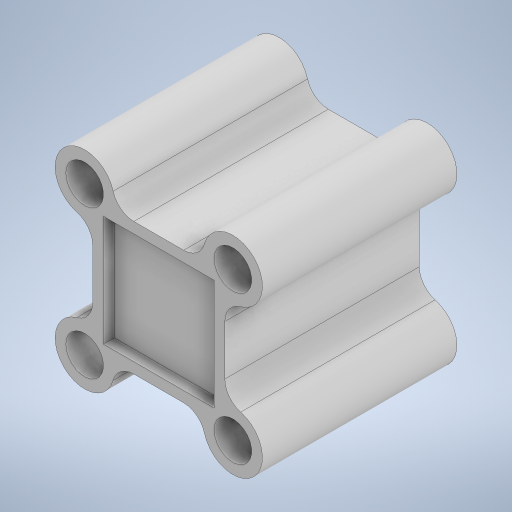
# Autodesk Inventor part: base_cube
Saved by Autodesk Inventor 2024.2 (Build 282272000, 272)
## iProperties
Created: 2021-12-13
Part Number: base_cube
Material: Generic
Document SubType Name: Modeling
Designer: magoo
Density: 1 g/cm^3
Appearance: Default
Description: 3D printing model
Author: magoo
Autodesk Inventor part; units mm, degrees
ref_plane "YZ Plane" through (0, 0, 0) normal (1, 0, 0) x (0, 1, 0)
ref_plane "XZ Plane" through (0, 0, 0) normal (0, 1, 0) x (-1, 0, 0)
ref_plane "XY Plane" through (0, 0, 0) normal (0, 0, 1) x (1, 0, 0)
sketch "Sketch1" plane through (0, 0, 0) normal (0, 0, 1) x (1, 0, 0)
  line L0 (6.15, -6.15) -> (-6.15, -6.15)
  line L1 (-6.15, -6.15) -> (-6.15, 6.15)
  line L2 (-6.15, 6.15) -> (6.15, 6.15)
  line L3 (6.15, 6.15) -> (6.15, -6.15)
  line L4 (6.15, -6.15) -> (-6.15, 6.15) construction
  line L5 (-6.15, -6.15) -> (6.15, 6.15) construction
  line L6 (5.15, -5.15) -> (-5.15, -5.15)
  line L7 (-5.15, -5.15) -> (-5.15, 5.15)
  line L8 (-5.15, 5.15) -> (5.15, 5.15)
  line L9 (5.15, 5.15) -> (5.15, -5.15)
  line L10 (5.15, -5.15) -> (-5.15, 5.15) construction
  line L11 (-5.15, -5.15) -> (5.15, 5.15) construction
  point P0 (0, 0)
  dimension "d0" = 12.3
  dimension "d1" = 12.3
  dimension "d2" = 10.3
  constraints: 24 end point, 4 midpoint, 4 parallel, 2 horizontal, 2 perpendicular, 1 point on line
  measures "d0" distance of L1.end L2.end
  measures "d1" distance of L0.end L1.end
  measures "d2" distance of L7.end L8.end
extrude "Extrusion1" add sketch "Sketch1" along normal blind 17.1 contours L6 L7 L8 L9
extrude "Extrusion2" add sketch "Sketch1" along normal blind 18.1
sketch "Sketch2" plane through (0, 0, 0) normal (0, 0, 1) x (1, 0, 0)
  line L0 (-6.15, 6.15) -> (-6.15, -6.15) construction
  line L1 (-6.15, 0) -> (6.15, 0)
  line L2 (6.15, -6.15) -> (6.15, 6.15) construction
  line L3 (6.15, 6.15) -> (-6.15, 6.15) construction
  line L4 (0, 6.15) -> (0, -6.15)
  line L5 (-6.15, -6.15) -> (6.15, -6.15) construction
  point P0 (0, 0)
  constraints: 4 end point, 4 midpoint
sketch "Sketch3" plane through (0, 0, 0) normal (0, 0, 1) x (1, 0, 0)
  circle A0 centre (-6.9, 6.9) radius 1.75
  line L0 (-11.15, -11.15) -> (11.15, -11.15) construction
  line L1 (11.15, -11.15) -> (11.15, 11.15) construction
  line L2 (11.15, 11.15) -> (-11.15, 11.15) construction
  line L3 (-11.15, 11.15) -> (-11.15, -11.15) construction
  line L4 (-11.15, -11.15) -> (11.15, 11.15) construction
  line L5 (11.15, -11.15) -> (-11.15, 11.15) construction
  line L6 (-6.15, 6.15) -> (-6.15, -6.15) projected
  line L7 (6.15, 6.15) -> (-6.15, 6.15) projected
  line L8 (-5.15, 5.15) -> (5.15, 5.15) projected
  circle A1 centre (6.9, 6.9) radius 1.75
  circle A2 centre (-6.9, -6.9) radius 1.75
  circle A3 centre (6.9, -6.9) radius 1.75
  line L9 (5.15, -5.15) -> (-5.15, -5.15) projected
  circle A4 centre (-6.9, 6.9) radius 2.75
  circle A5 centre (6.9, 6.9) radius 2.75
  circle A6 centre (6.9, -6.9) radius 2.75
  circle A7 centre (-6.9, -6.9) radius 2.75
  line L10 (5.15, 5.15) -> (-5.15, 5.15) projected
  line L11 (-5.15, 5.15) -> (-5.15, -5.15) projected
  line L12 (-5.15, -5.15) -> (5.15, -5.15) projected
  line L13 (5.15, -5.15) -> (5.15, 5.15) projected
  point P0 (0, 0)
  point P1 (0, 0)
  point P2 (-4.2542, 6.15)
  point P3 (-6.15, 4.2542)
  point P4 (-5.3189, 6.15)
  point P5 (-6.15, 5.3189)
  point P6 (-4.7787, -5.15)
  point P7 (-5.15, -4.7787)
  point P8 (5.15, -4.7787)
  point P9 (4.7787, -5.15)
  point P10 (-5.15, 4.7787)
  point P11 (-4.7787, 5.15)
  point P12 (4.7787, 5.15)
  point P13 (5.15, 5.15)
  point P14 (5.15, 4.7787)
  dimension "d19" = 3.5
  dimension "d20" = 5
  dimension "d21" = 5
  dimension "d22" = 3.5
  dimension "d23" = 3.5
  dimension "d24" = 3.5
  dimension "d25" = 5.5
  dimension "d26" = 5.5
  dimension "d27" = 5.5
  dimension "d28" = 5.5
  constraints: 12 end point, 8 centre point, 5 coincident, 4 point on line, 4 tangent, 2 midpoint, 2 parallel, 1 horizontal, 1 perpendicular
  measures "d19" diameter of A0
  measures "d20" distance between parallel lines of L3 L6
  measures "d21" distance between parallel lines of L2 L7
  measures "d22" diameter of A1
  measures "d23" diameter of A3
  measures "d24" diameter of A2
  measures "d25" diameter of A4
  measures "d26" diameter of A5
  measures "d27" diameter of A7
  measures "d28" diameter of A6
extrude "Extrusion4" add sketch "Sketch3" along normal up to surface (18.1 mm away) contours A0 L7 L6 | A0 L6 A4 L7 | L6 L7 A0 | A0 L7 A4 L8 L11 L6 | A2 | A7 L11 L9 | A1 | A5 L13 L8 | L9 L13 A6 | A3 picked at (-4.5292, -7.2681) picked at (5.5596, 5.0279) picked at (4.9749, -5.6466)
extrude "Extrusion5" cut sketch "Sketch3" along normal up to next contours A0 L7 L6 | L6 L7 A0 | A2 | A1 | A3
fillet "Fillet1" radius 2 8 edges at (-4.2542, -6.15, 9.05) (-6.15, -4.2542, 9.05) (-6.15, 4.2542, 9.05) (-4.2542, 6.15, 9.05) (4.2542, 6.15, 9.05) (6.15, 4.2542, 9.05) (6.15, -4.2542, 9.05) (4.2542, -6.15, 9.05)
body "Solid1"
